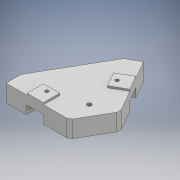
# Autodesk Inventor part: Delta Feet
Saved by Autodesk Inventor 2018 (Build 220112000, 112)
## iProperties
Created: 2018-03-30
Part Number: Delta Feet
Material: Generic
Document SubType Name: Modeling
Designer: elect
Density: 1 g/cm^3
Appearance: Default
Author: elect
Autodesk Inventor part; units mm, degrees
ref_plane "YZ Plane" through (0, 0, 0) normal (1, 0, 0) x (0, 1, 0)
ref_plane "XZ Plane" through (0, 0, 0) normal (0, 1, 0) x (-1, 0, 0)
ref_plane "XY Plane" through (0, 0, 0) normal (0, 0, 1) x (1, 0, 0)
sketch "Sketch1" plane through (0, 0, 0) normal (0, 0, 1) x (1, 0, 0)
  line L0 (-27.669, 1.4923) -> (-27.669, 15.9923)
  line L1 (-27.669, 15.9923) -> (-47.669, 15.9923)
  line L2 (-47.669, 15.9923) -> (-47.669, 1.4923)
  line L3 (4.7848, 57.9257) -> (-7.7725, 50.6757)
  line L4 (-7.7725, 50.6757) -> (-17.7732, 67.9973)
  line L5 (-17.7732, 67.9973) -> (-5.2158, 75.2473)
  circle A0 centre (-1.2464, 23.3799) radius 2.05
  line L6 (-47.669, 1.4923) -> (-67.669, 1.4923)
  line L7 (-27.669, 1.4923) -> (-0.5414, 1.7834)
  line L8 (4.7848, 57.9257) -> (18.3286, 34.4672)
  line L9 (-0.7095, 1.4923) -> (18.3286, 34.4672)
  line L10 (-15.2158, 92.5678) -> (-5.2158, 75.2473)
  line L11 (-47.669, 1.4923) -> (-67.669, 1.4923)
  line L12 (-67.669, 1.4923) -> (-67.669, 11.5002)
  line L13 (-47.669, 11.5) -> (-47.669, 1.4923)
  line L14 (-5.2158, 75.2473) -> (-15.2158, 92.5678)
  line L15 (-15.2158, 92.5678) -> (-23.5411, 87.7613)
  line L16 (-13.8463, 70.2645) -> (-5.2158, 75.2473)
  line L17 (-5.2158, 75.2473) -> (14.7842, 75.2473) construction
  line L18 (-23.5411, 87.7613) -> (-67.669, 11.5002)
  line L19 (18.3286, 34.4672) -> (22.6587, 36.9672)
  line L20 (-0.7095, 1.4923) -> (-0.7095, -3.5077)
  line L21 (-67.669, 1.4923) -> (-67.669, -3.5077)
  line L22 (-47.669, 1.4923) -> (-47.669, -3.5077)
  line L23 (-47.669, -3.5077) -> (-67.669, -3.5077)
  line L24 (-27.669, 1.4923) -> (-27.669, -3.5077)
  line L25 (-27.669, -3.5077) -> (-0.7095, -3.5077)
  line L26 (4.7848, 57.9257) -> (9.115, 60.4257)
  line L27 (9.115, 60.4257) -> (22.6587, 36.9672)
  line L28 (-15.2158, 92.5678) -> (-10.8857, 95.0678)
  line L29 (-5.2158, 75.2473) -> (-0.8857, 77.7473)
  line L30 (-0.8857, 77.7473) -> (-10.8857, 95.0678)
  line L31 (-23.5411, 87.7613) -> (-18.5411, 87.7613) construction
  line L32 (-0.7095, 1.4923) -> (3.6206, -1.0077)
  line L33 (-0.7095, 1.4923) -> (4.2905, 1.4923) construction
  line L34 (18.3286, 34.4672) -> (22.6587, 31.9672)
  line L35 (18.3286, 34.4672) -> (23.3286, 34.4672) construction
  line L36 (-67.669, 11.5002) -> (-71.9991, 14.0002)
  line L37 (-67.669, 11.5002) -> (-62.669, 11.5002) construction
  line L38 (-23.5411, 87.7613) -> (-27.8713, 90.261)
  line L39 (-27.8713, 90.261) -> (-71.9991, 14.0002)
  line L40 (3.6206, -1.0077) -> (22.6587, 31.9672)
  line L41 (-71.9991, 14.0002) -> (-71.9991, -3.5077)
  line L42 (-71.9991, -3.5077) -> (-67.669, -3.5077)
  line L43 (-10.8857, 95.0678) -> (-13.0507, 98.8177)
  line L44 (-13.0507, 98.8177) -> (-27.8713, 90.261)
  line L45 (22.6587, 31.9672) -> (22.6587, 36.9672)
  line L46 (-0.7095, -3.5077) -> (3.6206, -1.0077)
  point P0 (0, 0)
  point P1 (0, 0)
  dimension "d19" = 4.1
  dimension "d21" = 20
  dimension "d23" = 20
  dimension "d24" = 120
  dimension "d26" = 5
  dimension "d27" = 5
  dimension "d28" = 5
  dimension "d29" = 5
  dimension "d30" = 5
  dimension "d31" = 5
  dimension "d32" = 5
  dimension "d33" = 5
  dimension "d39" = 5
  dimension "d40" = 30
  dimension "d41" = 5
  dimension "d42" = 30
  dimension "d43" = 5
  dimension "d44" = 150
  dimension "d45" = 5
  dimension "d46" = 4.33
  dimension "d55" = 90
  dimension "d56" = 120
  dimension "d57" = 90
  dimension "d58" = 90
  constraints: 94 end point, 9 perpendicular, 6 horizontal, 5 vertical, 4 equal length, 3 parallel, 3 point on line, 2 collinear, 1 centre point
  measures "d19" diameter of A0
  measures "d21" distance of L12.end L13.start
  measures "d23" distance of L10.start L5.end
  measures "d24" angle of L17 L14
  measures "d26" distance of L8.end L19.end
  measures "d27" distance of L9.start L20.end
  measures "d28" distance of L6.end L21.end
  measures "d29" distance of L2.end L22.end
  measures "d30" distance of L0.start L24.end
  measures "d31" distance of L3.start L26.end
  measures "d32" distance of L10.start L28.end
  measures "d33" distance of L5.end L29.end
  measures "d39" distance of L9.start L32.end
  measures "d40" angle of L32 L33
  measures "d41" distance of L8.end L34.end
  measures "d42" angle of L34 L35
  measures "d43" distance of L12.end L36.end
  measures "d44" angle of L37 L36
  measures "d45" distance of L15.end L38.end
  measures "d46" distance of L28.end L43.end
  measures "d55" angle of L3 L8
  measures "d56" angle of L9 L8
  measures "d57" angle of L5 L4
  measures "d58" angle of L10 L5
extrude "Extrusion1" add sketch "Sketch1" along normal blind 20
sketch "Sketch4" plane through (-27.669, -3.5077, 0) normal (-1, 0, 0) x (0, 0, 1)
  line L0 (20, 19.5) -> (20, 0) projected
  line L1 (0, 19.5) -> (20, 19.5) projected
  line L2 (20, 0) -> (18, 0)
  line L3 (18, 0) -> (18, 19.5)
  line L4 (18, 19.5) -> (20, 19.5)
  line L5 (20, 19.5) -> (20, 0)
  point P0 (0, 3.5077)
  dimension "d59" = 2
  constraints: 8 end point, 2 parallel, 1 horizontal, 1 perpendicular, 1 point on line
  measures "d59" distance of L3.end L4.end
extrude "Extrusion4" add sketch "Sketch4" along normal blind 20
sketch "Sketch5" plane through (-0.8857, 77.7473, 0) normal (0.5, -0.8660254, 0) x (0.8660254, 0.5, 0)
  line L0 (0, 0) -> (0, 20) projected
  line L1 (0, 20) -> (-19.5, 20)
  line L2 (-19.5, 20) -> (-19.5, 18)
  line L3 (-19.5, 18) -> (0, 18)
  line L4 (0, 18) -> (0, 20)
  point P0 (-38.1066, 0)
  dimension "d62" = 19.5
  dimension "d63" = 2
  constraints: 8 end point, 2 parallel, 1 horizontal, 1 perpendicular
  measures "d62" distance of L3.end L2.end
  measures "d63" distance of L2.end L1.end
extrude "Extrusion5" add sketch "Sketch5" along normal blind 21
sketch "Sketch7" plane through (0, 0, 0) normal (0, 0, -1) x (-1, 0, 0)
  line L0 (0, 0) -> (0, 23.3799)
  circle A0 centre (1.2464, 23.3799) radius 2.05 projected
  line L1 (0, 23.3799) -> (1.2464, 23.3799)
  constraints: 4 end point, 1 perpendicular, 1 vertical
hole "Hole1" at (-1.2464, 23.3799, 0) direction (0, 0, 1) diameter 5 end through all counterbore diameter 8.2 counterbore depth 10
sketch "Sketch8" plane through (-0.8857, 77.7473, 18) normal (0, 0, -1) x (-0.8660254, -0.5, 0)
  line L0 (0, 0) -> (0, -20.0013) projected
  line L1 (19.5, -20.0013) -> (0, -20.0013) projected
  line L2 (0, 0) -> (19.5, 0)
  line L3 (19.5, 0) -> (19.5, -20.0013)
  line L4 (19.5, -20.0013) -> (0, -20.0013)
  line L5 (0, -20.0013) -> (0, 0)
  point P0 (38.1066, -67.774)
  constraints: 8 end point, 2 parallel, 1 horizontal, 1 perpendicular
extrude "Extrusion6" add sketch "Sketch8" along normal blind 8 and the other way blind 4
sketch "Sketch9" plane through (-27.669, -3.5077, 18) normal (0, 0, -1) x (-1, 0, 0)
  line L0 (20, 0) -> (20, 19.5) projected
  line L1 (0, 0) -> (20, 0)
  line L2 (20, 0) -> (20, 19.5)
  line L3 (20, 19.5) -> (0, 19.5)
  line L4 (0, 19.5) -> (0, 0)
  point P0 (-27.669, 3.5077)
  constraints: 8 end point, 2 parallel, 1 horizontal, 1 perpendicular
extrude "Extrusion7" add sketch "Sketch9" along normal blind 8 and the other way blind 4
sketch "Sketch10" plane through (-0.8857, 77.7473, 22) normal (0, 0, 1) x (0.8660254, 0.5, 0)
  line L0 (0, 0) -> (-19.5, 0) projected
  line L1 (-19.5, -20.0013) -> (0, -20.0013) projected
  line L2 (0, 0) -> (-5, 0)
  line L3 (-5, 0) -> (-5, -20.0013)
  line L4 (-5, -20.0013) -> (0, -20.0013)
  line L5 (0, -20.0013) -> (0, 0)
  line L6 (-5, -20.0013) -> (-13.5, -20.0013)
  line L7 (-13.5, -20.0013) -> (-13.5, -10.0013)
  line L8 (-13.5, -10.0013) -> (-5, -10.0013)
  line L9 (-5, -10.0013) -> (-5, -20.0013)
  point P0 (-38.1066, -67.774)
  dimension "d81" = 5
  dimension "d82" = 8.5
  dimension "d83" = 10
  constraints: 16 end point, 4 parallel, 2 horizontal, 2 perpendicular, 1 point on line
  measures "d81" distance of L4.end L3.end
  measures "d82" distance of L7.end L8.end
  measures "d83" distance of L6.end L7.end
hole "Hole2" at (-7.5764, 62.3359, 22) direction (0, 0, -1) diameter 4 end through all
sketch "Sketch11" plane through (-27.669, -3.5077, 22) normal (0, 0, 1) x (1, 0, 0)
  line L0 (-20, 0) -> (0, 0) projected
  line L1 (0, 0) -> (-20, 0)
  line L2 (-20, 0) -> (-20, 5)
  line L3 (-20, 5) -> (0, 5)
  line L4 (0, 5) -> (0, 0)
  line L5 (-20, 5) -> (-10, 5)
  line L6 (-10, 5) -> (-10, 13.5)
  line L7 (-10, 13.5) -> (-20, 13.5)
  line L8 (-20, 13.5) -> (-20, 5)
  point P0 (27.669, 3.5077)
  dimension "d91" = 20
  dimension "d92" = 5
  dimension "d93" = 10
  dimension "d101" = 8.5
  constraints: 16 end point, 4 parallel, 2 horizontal, 2 perpendicular
  measures "d91" distance of L2.end L3.end
  measures "d92" distance of L1.end L2.end
  measures "d93" distance of L7.end L6.end
  measures "d101" distance of L5.end L6.end
hole "Hole3" at (-37.669, 9.9923, 22) direction (0, 0, -1) diameter 4 end through all
sketch "Sketch12" plane through (9.115, 60.4257, 20) normal (0.5, -0.8660254, 0) x (0.8660254, 0.5, 0)
  line L0 (0, 0) -> (-19.5, 0)
  line L1 (-19.5, 0) -> (-19.5, 2)
  line L2 (-19.5, 2) -> (0, 2)
  line L3 (0, 2) -> (0, 0)
  point P0 (-38.1066, -20)
  constraints: 8 end point, 2 parallel, 1 horizontal, 1 perpendicular
extrude "Extrusion8" cut sketch "Sketch12" against normal blind 0.4
sketch "Sketch13" plane through (-17.7732, 67.9973, 22) normal (-0.5, 0.8660254, 0) x (0.8660254, 0.5, 0)
  line L0 (19.5, 0) -> (0, 0) projected
  line L1 (19.5, 2) -> (19.5, 0) projected
  line L2 (0, 0) -> (19.5, 0)
  line L3 (19.5, 0) -> (19.5, 2)
  line L4 (19.5, 2) -> (0, 2)
  line L5 (0, 2) -> (0, 0)
  point P0 (-18.6066, 22)
  constraints: 8 end point, 2 parallel, 1 horizontal, 1 perpendicular
extrude "Extrusion9" cut sketch "Sketch13" against normal blind 0.4
sketch "Sketch14" plane through (-7.9725, 51.0221, 20) normal (-0.8660254, -0.5, 0) x (0, 0, 1)
  line L0 (0, 0) -> (0, 19.2013) projected
  line L1 (2, 19.2013) -> (2, 0) projected
  line L2 (0, 0) -> (2, 0)
  line L3 (2, 0) -> (2, 19.2013)
  line L4 (2, 19.2013) -> (0, 19.2013)
  line L5 (0, 19.2013) -> (0, 0)
  point P0 (-20, -48.1727)
  constraints: 8 end point, 2 parallel, 1 horizontal, 1 perpendicular
extrude "Extrusion10" cut sketch "Sketch14" against normal blind 0.4
sketch "Sketch15" plane through (-47.669, -3.5077, 20) normal (-1, 0, 0) x (0, 0, 1)
  line L0 (0, 0) -> (2, 0)
  line L1 (2, 0) -> (2, 19.5)
  line L2 (2, 19.5) -> (0, 19.5)
  line L3 (0, 19.5) -> (0, 0)
  point P0 (-20, 3.5077)
  constraints: 8 end point, 2 parallel, 1 horizontal, 1 perpendicular
extrude "Extrusion11" cut sketch "Sketch15" against normal blind 0.4
sketch "Sketch16" plane through (-27.669, -3.5077, 20) normal (1, 0, 0) x (0, 0, -1)
  line L0 (0, 19.5) -> (0, 0) projected
  line L1 (-2, 0) -> (-2, 19.5) projected
  line L2 (0, 0) -> (-2, 0)
  line L3 (-2, 0) -> (-2, 19.5)
  line L4 (-2, 19.5) -> (0, 19.5)
  line L5 (0, 19.5) -> (0, 0)
  point P0 (20, 3.5077)
  constraints: 8 end point, 2 parallel, 1 horizontal, 1 perpendicular
extrude "Extrusion12" cut sketch "Sketch16" against normal blind 0.4
sketch "Sketch17" plane through (-47.269, 15.9923, 22) normal (0, 1, 0) x (1, 0, 0)
  line L0 (19.2, 0) -> (0, 0) projected
  line L1 (0, 2) -> (19.2, 2)
  line L2 (19.2, 2) -> (19.2, 0)
  line L3 (19.2, 0) -> (0, 0)
  line L4 (0, 0) -> (0, 2)
  point P0 (47.269, 22)
  constraints: 8 end point, 2 parallel, 1 horizontal, 1 perpendicular
extrude "Extrusion13" cut sketch "Sketch17" against normal blind 0.4
body "Solid1"
